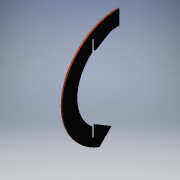
# Autodesk Inventor part: 19in inner coil
Saved by Autodesk Inventor 2016 (Build 200138000, 138)
## iProperties
Created: 2016-01-31
Part Number: 19in inner coil
Material: Acetal Resin, Black
Document SubType Name: Modeling
Designer: Scott
Density: 1.425 g/cm^3
Appearance: Smooth - Black
Mass: 370.188 g
Surface Area: 952.299 cm^2
Volume: 259.781 cm^3
Author: Scott
Autodesk Inventor part; units mm, degrees
ref_plane "YZ Plane" through (0, 0, 0) normal (1, 0, 0) x (0, 1, 0)
ref_plane "XZ Plane" through (0, 0, 0) normal (0, 1, 0) x (-1, 0, 0)
ref_plane "XY Plane" through (0, 0, 0) normal (0, 0, 1) x (1, 0, 0)
sketch "Sketch1" plane through (0, 0, 0) normal (1, 0, 0) x (0, 1, 0)
  arc A0 (241.3, 0) -> (-241.3, 0) centre (0, 0) ccw
  arc A1 (177.8, 0) -> (-177.8, 0) centre (0, 0) ccw
  line L0 (-177.8, 0) -> (-241.3, 0)
  circle A2 centre (221.8868, 12.7) radius 3.175
  circle A3 centre (0, 0) radius 222.25 construction
  circle A4 centre (218.9887, 37.9341) radius 3.175
  circle A5 centre (213.2304, 62.6728) radius 3.175
  circle A6 centre (0, 0) radius 196.85 construction
  circle A7 centre (186.6826, 62.4463) radius 3.175
  circle A8 centre (193.1693, 37.8886) radius 3.175
  circle A9 centre (196.4399, 12.7) radius 3.175
  line L1 (0, 0) -> (360.6027, 0)
  line L2 (360.6027, 0) -> (-412.5993, 0)
  line L3 (0, 0) -> (0, -65.1131)
  circle A10 centre (-221.8868, 12.7) radius 3.175
  circle A11 centre (-218.9887, 37.9341) radius 3.175
  circle A12 centre (-213.2304, 62.6728) radius 3.175
  circle A13 centre (-186.6826, 62.4463) radius 3.175
  circle A14 centre (-193.1693, 37.8886) radius 3.175
  circle A15 centre (-196.4399, 12.7) radius 3.175
  line L4 (0, 0) -> (205.1572, 205.1572)
  line L5 (0, 0) -> (-243.5425, 243.5425)
  circle A16 centre (-12.7, 221.8868) radius 3.175
  circle A17 centre (-37.9341, 218.9887) radius 3.175
  circle A18 centre (-62.6728, 213.2304) radius 3.175
  circle A19 centre (-62.4463, 186.6826) radius 3.175
  circle A20 centre (-37.8886, 193.1693) radius 3.175
  circle A21 centre (-12.7, 196.4399) radius 3.175
  circle A22 centre (12.7, 221.8868) radius 3.175
  circle A23 centre (37.9341, 218.9887) radius 3.175
  circle A24 centre (62.6728, 213.2304) radius 3.175
  circle A25 centre (62.4463, 186.6826) radius 3.175
  circle A26 centre (37.8886, 193.1693) radius 3.175
  circle A27 centre (12.7, 196.4399) radius 3.175
  line L6 (241.3, 0) -> (177.8, 0)
  dimension "d0" = 482.6
  dimension "d1" = 355.6
  dimension "d2" = 6.35
  dimension "d3" = 444.5
  dimension "d4" = 6.35
  dimension "d5" = 6.35
  dimension "d6" = 25.4
  dimension "d7" = 25.4
  dimension "d8" = 393.7
  dimension "d9" = 6.35
  dimension "d10" = 6.35
  dimension "d11" = 6.35
  dimension "d13" = 12.7
  dimension "d14" = 12.7
  dimension "d15" = 25.4
  dimension "d16" = 25.4
  dimension "d17" = 45
  dimension "d18" = 45
  constraints: 28 centre point, 18 symmetric about line, 14 end point, 10 point on circle, 4 coincident, 3 horizontal, 1 point on line, 1 vertical, 18 other
  measures "d0" diameter of A0
  measures "d1" diameter of A1
  measures "d2" diameter of A2
  measures "d3" diameter of A3
  measures "d4" diameter of A5
  measures "d5" diameter of A4
  measures "d6" distance of A2.centre A4.centre
  measures "d7" distance of A4.centre A5.centre
  measures "d8" diameter of A6
  measures "d9" diameter of A9
  measures "d10" diameter of A8
  measures "d11" diameter of A7
  measures "d13" distance from line of L1 A2.centre
  measures "d14" distance from line of L1 A9.centre
  measures "d15" distance of A9.centre A8.centre
  measures "d16" distance of A8.centre A7.centre
  measures "d17" angle of L1 L4
  measures "d18" angle of L2 L5
extrude "Extrusion1" add sketch "Sketch1" along normal blind 6.35 contours L1 A1 L4 A0 | L4 A1 L5 A0 | L5 A1 L0 A0
sketch "Sketch2" plane through (6.35, 0, 0) normal (1, 0, 0) x (0, 0, -1)
  line L0 (-101.6, 183.162) -> (-101.6, 145.9119) projected
  arc A0 (101.6, 145.9119) -> (-101.6, 145.9119) centre (0, 0) ccw projected
  line L1 (101.6, 145.9119) -> (101.6, 183.162) projected
  line L2 (101.6, 183.162) -> (114.3, 183.162) projected
  line L3 (114.3, 183.162) -> (114.3, 136.1923) projected
  arc A1 (177.8, 0) -> (114.3, 136.1923) centre (0, 0) ccw projected
  line L4 (177.8, 0) -> (254, 0) projected
  arc A2 (254, 0) -> (50.0287, 249.0244) centre (0, 0) ccw projected
  arc A3 (36.5783, 256.4729) -> (50.0287, 249.0244) centre (55.0316, 273.9268) ccw projected
  arc A4 (36.5783, 256.4729) -> (-36.5783, 256.4729) centre (0, 221.8757) ccw projected
  arc A5 (-50.0287, 249.0244) -> (-36.5783, 256.4729) centre (-55.0316, 273.9268) ccw projected
  arc A6 (-50.0287, 249.0244) -> (-254, 0) centre (0, 0) ccw projected
  line L5 (-254, 0) -> (-177.8, 0) projected
  arc A7 (-114.3, 136.1923) -> (-177.8, 0) centre (0, 0) ccw projected
  line L6 (-114.3, 136.1923) -> (-114.3, 183.162) projected
  line L7 (-114.3, 183.162) -> (-101.6, 183.162) projected
  circle A8 centre (-196.4399, 12.7) radius 3.302 projected
  circle A9 centre (-218.9887, 37.9341) radius 3.302 projected
  circle A10 centre (-186.6826, 62.4463) radius 3.302 projected
  circle A11 centre (-62.4463, 186.6826) radius 3.302 projected
  circle A12 centre (-37.9341, 218.9887) radius 3.302 projected
  circle A13 centre (-12.7, 196.4399) radius 3.302 projected
  circle A14 centre (12.7, 221.8868) radius 3.302 projected
  circle A15 centre (37.8886, 193.1693) radius 3.302 projected
  circle A16 centre (62.6728, 213.2304) radius 3.302 projected
  circle A17 centre (196.4399, 12.7) radius 3.302 projected
  circle A18 centre (193.1693, 37.8886) radius 3.302 projected
  circle A19 centre (186.6826, 62.4463) radius 3.302 projected
  circle A20 centre (213.2304, 62.6728) radius 3.302 projected
  circle A21 centre (218.9887, 37.9341) radius 3.302 projected
  circle A22 centre (221.8868, 12.7) radius 3.302 projected
  circle A23 centre (62.4463, 186.6826) radius 3.302 projected
  circle A24 centre (37.9341, 218.9887) radius 3.302 projected
  circle A25 centre (12.7, 196.4399) radius 3.302 projected
  circle A26 centre (-12.7, 221.8868) radius 3.302 projected
  circle A27 centre (-37.8886, 193.1693) radius 3.302 projected
  circle A28 centre (-62.6728, 213.2304) radius 3.302 projected
  circle A29 centre (-213.2304, 62.6728) radius 3.302 projected
  circle A30 centre (-193.1693, 37.8886) radius 3.302 projected
  circle A31 centre (-221.8868, 12.7) radius 3.302 projected
  circle A32 centre (0, 259.6856) radius 3.302 projected
  line L8 (0, 0) -> (-75.0645, 0)
  line L9 (-114.3, 183.162) -> (-101.6, 183.162)
  line L10 (-101.6, 183.162) -> (-101.6, 75.1342)
  line L11 (-101.6, 75.1342) -> (-114.3, 75.1342)
  line L12 (-114.3, 75.1342) -> (-114.3, 183.162)
  line L13 (-114.3, -136.1923) -> (-114.3, -183.162)
  line L14 (-114.3, -183.162) -> (-101.6, -183.162)
  line L15 (-101.6, -183.162) -> (-101.6, -75.1342)
  line L16 (-101.6, -75.1342) -> (-114.3, -75.1342)
  line L17 (-114.3, -75.1342) -> (-114.3, -183.162)
  line L18 (-114.3, -183.162) -> (-101.6, -183.162)
  line L19 (-101.6, -183.162) -> (-101.6, -75.1342)
  line L20 (-101.6, -75.1342) -> (-114.3, -75.1342)
  line L21 (-114.3, -75.1342) -> (-114.3, -183.162)
  point P0 (0, 0)
  constraints: 24 end point, 6 symmetric about line, 4 parallel, 3 horizontal, 2 perpendicular
extrude "Extrusion2" cut sketch "Sketch2" against normal blind 25.4 contours L0 L10 L11 L12 L6 L7 | L17 L16 L15 L14 L13
sketch "Sketch3" plane through (6.35, 0, 0) normal (1, 0, 0) x (0, 0, -1)
  line L0 (-101.6, 183.162) -> (-101.6, 136.1923) projected
  line L1 (-101.6, 136.1923) -> (-38.1, 173.6699) projected
  arc A0 (38.1, 173.6699) -> (-38.1, 173.6699) centre (0, 0) ccw projected
  line L2 (38.1, 173.6699) -> (101.6, 136.1923) projected
  line L3 (101.6, 136.1923) -> (101.6, 183.162) projected
  line L4 (101.6, 183.162) -> (114.3, 183.162) projected
  line L5 (114.3, 183.162) -> (114.3, 136.1923) projected
  arc A1 (177.8, 0) -> (114.3, 136.1923) centre (0, 0) ccw projected
  line L6 (177.8, 0) -> (254, 0) projected
  arc A2 (254, 0) -> (50.0287, 249.0244) centre (0, 0) ccw projected
  arc A3 (36.5783, 256.4729) -> (50.0287, 249.0244) centre (55.0316, 273.9268) ccw projected
  arc A4 (36.5783, 256.4729) -> (-36.5783, 256.4729) centre (0, 221.8757) ccw projected
  arc A5 (-50.0287, 249.0244) -> (-36.5783, 256.4729) centre (-55.0316, 273.9268) ccw projected
  arc A6 (-50.0287, 249.0244) -> (-254, 0) centre (0, 0) ccw projected
  line L7 (-254, 0) -> (-177.8, 0) projected
  arc A7 (-114.3, 136.1923) -> (-177.8, 0) centre (0, 0) ccw projected
  line L8 (-114.3, 136.1923) -> (-114.3, 183.162) projected
  line L9 (-114.3, 183.162) -> (-101.6, 183.162) projected
  circle A8 centre (-196.4399, 12.7) radius 3.302 projected
  circle A9 centre (-218.9887, 37.9341) radius 3.302 projected
  circle A10 centre (-186.6826, 62.4463) radius 3.302 projected
  circle A11 centre (-62.4463, 186.6826) radius 3.302 projected
  circle A12 centre (-37.9341, 218.9887) radius 3.302 projected
  circle A13 centre (-12.7, 196.4399) radius 3.302 projected
  circle A14 centre (12.7, 221.8868) radius 3.302 projected
  circle A15 centre (37.8886, 193.1693) radius 3.302 projected
  circle A16 centre (62.6728, 213.2304) radius 3.302 projected
  circle A17 centre (196.4399, 12.7) radius 3.302 projected
  circle A18 centre (193.1693, 37.8886) radius 3.302 projected
  circle A19 centre (186.6826, 62.4463) radius 3.302 projected
  circle A20 centre (213.2304, 62.6728) radius 3.302 projected
  circle A21 centre (218.9887, 37.9341) radius 3.302 projected
  circle A22 centre (221.8868, 12.7) radius 3.302 projected
  circle A23 centre (62.4463, 186.6826) radius 3.302 projected
  circle A24 centre (37.9341, 218.9887) radius 3.302 projected
  circle A25 centre (12.7, 196.4399) radius 3.302 projected
  circle A26 centre (-12.7, 221.8868) radius 3.302 projected
  circle A27 centre (-37.8886, 193.1693) radius 3.302 projected
  circle A28 centre (-62.6728, 213.2304) radius 3.302 projected
  circle A29 centre (-213.2304, 62.6728) radius 3.302 projected
  circle A30 centre (-193.1693, 37.8886) radius 3.302 projected
  circle A31 centre (-221.8868, 12.7) radius 3.302 projected
  circle A32 centre (0, 259.6856) radius 3.302 projected
  line L10 (0, 0) -> (-50.0287, 0)
  arc A33 (0, 177.8) -> (-101.6, 145.9119) centre (0, 0) ccw projected
  arc A34 (-38.1, 173.6699) -> (-101.6, 145.9119) centre (0, 0) ccw
  line L11 (-101.6, -145.9119) -> (-101.6, -183.162) projected
  line L12 (-101.6, -183.162) -> (-114.3, -183.162) projected
  line L13 (-114.3, -183.162) -> (-114.3, -136.1923) projected
  arc A35 (-177.8, 0) -> (-114.3, -136.1923) centre (0, 0) ccw projected
  line L14 (-177.8, 0) -> (-254, 0) projected
  line L15 (-254, 0) -> (-254, -254) projected
  line L16 (-254, -254) -> (254, -254) projected
  line L17 (254, -254) -> (254, 0) projected
  line L18 (254, 0) -> (177.8, 0) projected
  arc A36 (114.3, -136.1923) -> (177.8, 0) centre (0, 0) ccw projected
  line L19 (114.3, -136.1923) -> (114.3, -183.162) projected
  line L20 (114.3, -183.162) -> (101.6, -183.162) projected
  line L21 (101.6, -183.162) -> (101.6, -145.9119) projected
  arc A37 (-101.6, -145.9119) -> (101.6, -145.9119) centre (0, 0) ccw projected
  circle A38 centre (221.8868, -12.7) radius 3.302 projected
  circle A39 centre (193.1693, -37.8886) radius 3.302 projected
  circle A40 centre (213.2304, -62.6728) radius 3.302 projected
  circle A41 centre (62.4463, -186.6826) radius 3.302 projected
  circle A42 centre (37.9341, -218.9887) radius 3.302 projected
  circle A43 centre (12.7, -221.8868) radius 3.302 projected
  circle A44 centre (-12.7, -221.8868) radius 3.302 projected
  circle A45 centre (-37.9341, -218.9887) radius 3.302 projected
  circle A46 centre (-62.6728, -213.2304) radius 3.302 projected
  circle A47 centre (-186.6826, -62.4463) radius 3.302 projected
  circle A48 centre (-218.9887, -37.9341) radius 3.302 projected
  circle A49 centre (-196.4399, -12.7) radius 3.302 projected
  circle A50 centre (-221.8868, -12.7) radius 3.302 projected
  circle A51 centre (-193.1693, -37.8886) radius 3.302 projected
  circle A52 centre (-213.2304, -62.6728) radius 3.302 projected
  circle A53 centre (-62.4463, -186.6826) radius 3.302 projected
  circle A54 centre (-37.8886, -193.1693) radius 3.302 projected
  circle A55 centre (-12.7, -196.4399) radius 3.302 projected
  circle A56 centre (12.7, -196.4399) radius 3.302 projected
  circle A57 centre (37.8886, -193.1693) radius 3.302 projected
  circle A58 centre (62.6728, -213.2304) radius 3.302 projected
  circle A59 centre (186.6826, -62.4463) radius 3.302 projected
  circle A60 centre (218.9887, -37.9341) radius 3.302 projected
  circle A61 centre (196.4399, -12.7) radius 3.302 projected
  circle A62 centre (-215.9, -215.9) radius 3.302 projected
  circle A63 centre (215.9, -215.9) radius 3.302 projected
  line L22 (-101.6, -136.1923) -> (-38.1, -173.6699)
  line L23 (-101.6, -183.162) -> (-101.6, -145.9119) projected
  line L24 (-101.6, -136.1923) -> (-101.6, -145.9119)
  arc A64 (-101.6, -145.9119) -> (0, -177.8) centre (0, 0) ccw projected
  arc A65 (-101.6, -145.9119) -> (-38.1, -173.6699) centre (0, 0) ccw
  constraints: 5 point on circle, 4 end point, 2 centre point, 2 symmetric about line, 1 concentric, 1 horizontal, 1 point on line, 1 vertical
extrude "Extrusion3" add sketch "Sketch3" against normal blind 6.35 contours A33 L1 L0 | L24 L22 A37
body "Solid1"
